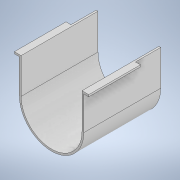
# Autodesk Inventor part: TapaEje
Saved by Autodesk Inventor 2020 (Build 240168000, 168)
## iProperties
Created: 2019-11-12
Part Number: TapaEje
Material: Genérico
Document SubType Name: Modeling
Designer: Usuario
Density: 1 g/cm^3
Appearance: Valor por defecto
Author: Usuario
## iProperties of the stored document _3DPrint.ipt
Created: 2019-11-12
Part Number: _3DPrint
Material: Genérico
Document SubType Name: Modeling
Designer: Usuario
Density: 1 g/cm^3
Appearance: Valor por defecto
Author: Usuario
Autodesk Inventor part; units mm, degrees
ref_plane "YZ Plane" through (0, 0, 0) normal (1, 0, 0) x (0, 1, 0)
ref_plane "XZ Plane" through (0, 0, 0) normal (0, 1, 0) x (-1, 0, 0)
ref_plane "XY Plane" through (0, 0, 0) normal (0, 0, 1) x (1, 0, 0)
sketch "Boceto1" plane through (0, 0, 0) normal (0, 0, 1) x (1, 0, 0)
  arc A0 (-52.5, 0) -> (52.5, 0) centre (0, 0) ccw
  line L0 (-52.5, 0) -> (-52.5, 57.5)
  line L1 (-52.5, 57.5) -> (-49.5, 57.5)
  line L2 (52.5, 57.5) -> (52.5, 0)
  arc A1 (52.5, 0) -> (-52.5, 0) centre (0, 0) ccw construction
  line L3 (0, -52.5) -> (0, 57.5) construction
  line L4 (-49.5, 57.5) -> (-49.5, 0)
  arc A2 (-49.5, 0) -> (49.5, 0) centre (0, 0) ccw
  line L5 (49.5, 0) -> (49.5, 57.5)
  line L6 (49.5, 57.5) -> (-49.5, 57.5) construction
  line L7 (49.5, 57.5) -> (49.5, 57.5)
  line L8 (-49.5, 57.5) -> (-49.5, 57.5)
  line L9 (-49.5, 57.5) -> (0, 57.5) construction
  line L10 (0, 57.5) -> (49.5, 57.5) construction
  line L11 (49.5, 57.5) -> (52.5, 57.5)
  dimension "d0" = 105
  dimension "d2" = 110
  dimension "d3" = 3
  constraints: 24 end point, 9 perpendicular, 7 point on circle, 3 centre point, 2 point on line, 2 tangent, 2 vertical, 1 coincident, 1 collinear, 1 parallel, 2 other
  measures "d0" diameter of A0
  measures "d2" distance of L3.start L3.end
  measures "d3" distance between parallel lines of L0 L4
extrude "Extrusión1" add sketch "Boceto1" along normal blind 41
sketch "Boceto2" plane through (0, 0, 41) normal (0, 0, 1) x (1, 0, 0)
  line L0 (49.5, 57.5) -> (49.5, 0) projected
  arc A0 (-49.5, 0) -> (49.5, 0) centre (0, 0) ccw projected
  line L1 (-49.5, 0) -> (-49.5, 57.5) projected
  line L2 (-49.5, 57.5) -> (-52.5, 57.5) projected
  line L3 (-52.5, 57.5) -> (-52.5, 0) projected
  arc A1 (-52.5, 0) -> (52.5, 0) centre (0, 0) ccw projected
  line L4 (52.5, 0) -> (52.5, 57.5) projected
  line L5 (52.5, 57.5) -> (49.5, 57.5) projected
  line L6 (-49.5, 57.5) -> (-52.5, 57.5) projected
  line L7 (-52.5, 57.5) -> (-60.5, 57.5)
  line L8 (-60.5, 57.5) -> (-60.5, 54.5)
  line L9 (-60.5, 54.5) -> (-52.5, 54.5)
  line L10 (-52.5, 54.5) -> (-52.5, 57.5)
  line L11 (52.5, 57.5) -> (49.5, 57.5) projected
  line L12 (52.5, 57.5) -> (60.5, 57.5)
  line L13 (60.5, 57.5) -> (60.5, 54.5)
  line L14 (60.5, 54.5) -> (52.5, 54.5)
  line L15 (52.5, 54.5) -> (52.5, 57.5)
  dimension "d6" = 8
  dimension "d7" = 3
  dimension "d8" = 8
  dimension "d9" = 3
  constraints: 16 end point, 4 parallel, 2 horizontal, 2 perpendicular
  measures "d6" distance of L2.end L7.end
  measures "d7" distance of L7.end L8.end
  measures "d8" distance of L4.end L12.end
  measures "d9" distance of L12.end L13.end
extrude "Extrusión2" add sketch "Boceto2" along normal blind 84
